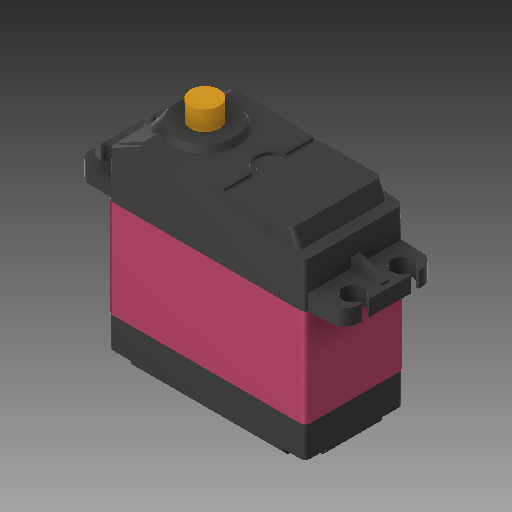
# Autodesk Inventor part: DS3218MG
Saved by Autodesk Inventor 2019.3 (Build 233278000, 278)
## iProperties
Created: 2019-03-07
Part Number: DS3218MG
Material: アルミニウム 6061
Document SubType Name: Modeling
Designer: TA
Density: 2.7 g/cm^3
Appearance: アルミニウム - フラット
Author: TA
Autodesk Inventor part; units mm, degrees
sketch "スケッチ1" plane through (0, 0, 0) normal (0, 1, 0) x (-1, 0, 0)
  line L0 (0, 0) -> (-40.06, 0)
  line L1 (-40.06, 0) -> (-40.06, -20)
  line L2 (-40.06, -20) -> (0, -20)
  line L3 (0, -20) -> (0, 0)
  dimension "d0" = 40.06
  dimension "d1" = 20
  constraints: 8 end point, 2 parallel, 1 horizontal, 1 perpendicular
  measures "d0" distance of L2.end L1.end
  measures "d1" distance of L1.end L0.end
ref_plane "作業平面1" through (0, 7.8, 0) normal (0, 1, 0) x (-1, 0, 0)
sketch "スケッチ2" plane through (0, 7.8, 0) normal (0, 1, 0) x (-1, 0, 0)
  line L0 (0.07, -20.1) -> (-40.13, -20.1)
  line L1 (-40.13, -20.1) -> (-40.13, 0.1)
  line L2 (-40.13, 0.1) -> (0.07, 0.1)
  line L3 (0.07, 0.1) -> (0.07, -20.1)
  line L4 (-40.06, -20) -> (0, -20) construction
  line L5 (0, -20) -> (0, 0) construction
  line L6 (0, 0) -> (-40.06, 0) construction
  line L7 (-40.06, 0) -> (-40.06, -20) construction
  dimension "d3" = 20.2
  dimension "d5" = 0.1
  dimension "d6" = 40.2
  dimension "d7" = 0.07
  constraints: 8 end point, 2 parallel, 1 horizontal, 1 perpendicular
  measures "d3" distance of L0.end L1.end
  measures "d5" distance between parallel lines of L0 L4
  measures "d6" distance of L1.end L2.end
  measures "d7" distance between parallel lines of L3 L5
loft "ロフト1" add profiles "スケッチ1", "スケッチ2"
fillet "フィレット2" radius 1 4 edges at (-0.035, 3.9, 0.05) (40.095, 3.9, 0.05) (40.095, 3.9, -20.05) (-0.035, 3.9, -20.05)
sketch "スケッチ4" plane through (0.9999, 0, -20) normal (0, -1, 0) x (1, 0, 0)
  line L0 (-1.0699, 15.5) -> (3.5301, 15.5)
  line L1 (3.5301, 15.5) -> (3.5301, 20.1)
  ellipse E0 centre (-0.0699, 19.0999) end of major axis (-0.6434, 19.9193) minor radius 1 (-0.07, 20.1) -> (-1.0699, 19.1) ccw projected
  line L2 (-0.07, 20.1) -> (38.1301, 20.1) projected
  line L3 (-1.0699, 0.9) -> (-1.0699, 19.1) projected
  point P0 (-0.9999, 20)
  dimension "d16" = 4.6
  dimension "d17" = 4.6
  constraints: 4 end point, 2 point on line, 1 perpendicular, 1 vertical, 1 other
  measures "d16" distance of L0.end L1.end
  measures "d17" distance between parallel lines of L3 L1
extrude "押し出し1" cut sketch "スケッチ4" against normal blind 1.5
fillet "フィレット3" radius 1.5 1 edges at (4.53, 0.75, -4.5)
ref_plane "作業平面2" through (0.9299, -780, -10) normal (0, 0, 1) x (-1, 0, 0)
ref_plane "作業平面3" through (20.03, -2231.9143, -19.1) normal (-1, 0, 0) x (0, 0, -1)
mirror "ミラー1" about plane through (0.9299, -780, -10) normal (0, 0, 1) of "押し出し1"
mirror "ミラー2" about plane through (20.03, -2231.9143, -19.1) normal (-1, 0, 0) of "押し出し1", "ミラー1"
chamfer "面取り1" distance 1 angle 45 4 edges at (20.03, 0, 0) (0, 0, -10) (20.03, 0, -20) (40.06, 0, -10)
sketch "スケッチ5" plane through (0.9299, 7.8, 0.1) normal (0, 1, 0) x (1, 0, 0)
  ellipse E0 centre (0.0001, 19.1999) end of major axis (-0.5734, 20.0193) minor radius 1 (0, 20.2) -> (-0.9999, 19.2) ccw projected
  line L0 (-0.9999, 19.2) -> (-0.9999, 1) projected
  ellipse E1 centre (0.0001, 1.0001) end of major axis (-0.5734, 0.1807) minor radius 1 (-0.9999, 1) -> (0, 0) ccw projected
  line L1 (0, 0) -> (38.2001, 0) projected
  ellipse E2 centre (38.2, 1.0001) end of major axis (38.7736, 0.1807) minor radius 1 (38.2001, 0) -> (39.2001, 1) ccw projected
  line L2 (39.2001, 1) -> (39.2001, 19.2) projected
  ellipse E3 centre (38.2, 19.1999) end of major axis (38.7736, 20.0193) minor radius 1 (39.2001, 19.2) -> (38.2001, 20.2) ccw projected
  line L3 (38.2001, 20.2) -> (0, 20.2) projected
  point P0 (-0.9299, 0.1)
  constraints: 4 other
extrude "押し出し2" add sketch "スケッチ5" along normal blind 19.9 separate body
sketch "スケッチ6" plane through (0.9299, 27.7, 0.1) normal (0, 1, 0) x (1, 0, 0)
  ellipse E0 centre (0.0001, 19.1999) end of major axis (-0.5734, 20.0193) minor radius 1 (0, 20.2) -> (-0.9999, 19.2) ccw projected
  line L0 (-0.9999, 19.2) -> (-0.9999, 1) projected
  ellipse E1 centre (0.0001, 1.0001) end of major axis (-0.5734, 0.1807) minor radius 1 (-0.9999, 1) -> (0, 0) ccw projected
  line L1 (0, 0) -> (38.2001, 0) projected
  ellipse E2 centre (38.2, 1.0001) end of major axis (38.7736, 0.1807) minor radius 1 (38.2001, 0) -> (39.2001, 1) ccw projected
  line L2 (39.2001, 1) -> (39.2001, 19.2) projected
  ellipse E3 centre (38.2, 19.1999) end of major axis (38.7736, 20.0193) minor radius 1 (39.2001, 19.2) -> (38.2001, 20.2) ccw projected
  line L3 (38.2001, 20.2) -> (0, 20.2) projected
  point P0 (-0.9299, 0.1)
  constraints: 4 other
ref_plane "作業平面4" through (0.9299, 40.4, 0.1) normal (0, 1, 0) x (1, 0, 0)
sketch "スケッチ7" plane through (0.9299, 40.4, 0.1) normal (0, 1, 0) x (1, 0, 0)
  ellipse E0 centre (0.0001, 19.1999) end of major axis (-0.5734, 20.0193) minor radius 1 (0, 20.2) -> (-0.9999, 19.2) ccw projected
  line L0 (-0.9999, 19.2) -> (-0.9999, 1) construction
  ellipse E1 centre (0.0001, 1.0001) end of major axis (-0.5734, 0.1807) minor radius 1 (-0.9999, 1) -> (0, 0) ccw projected
  line L1 (0, 0) -> (38.2001, 0) construction
  ellipse E2 centre (38.2, 1.0001) end of major axis (38.7736, 0.1807) minor radius 1 (38.2001, 0) -> (39.2001, 1) ccw projected
  line L2 (39.2001, 1) -> (39.2001, 19.2) construction
  ellipse E3 centre (38.2, 19.1999) end of major axis (38.7736, 20.0193) minor radius 1 (39.2001, 19.2) -> (38.2001, 20.2) ccw projected
  line L3 (38.2001, 20.2) -> (0, 20.2) construction
  line L4 (0.1501, 20.025) -> (38.0501, 20.025)
  line L5 (39.0501, 19.025) -> (39.0501, 1.175)
  line L6 (38.0501, 0.175) -> (0.1501, 0.175)
  line L7 (-0.8499, 1.175) -> (-0.8499, 19.025)
  arc A0 (0.1501, 20.025) -> (-0.8499, 19.025) centre (0.1501, 19.025) ccw
  arc A1 (39.0501, 19.025) -> (38.0501, 20.025) centre (38.0501, 19.025) ccw
  arc A2 (-0.8499, 1.175) -> (0.1501, 0.175) centre (0.1501, 1.175) ccw
  arc A3 (38.0501, 0.175) -> (39.0501, 1.175) centre (38.0501, 1.175) ccw
  point P0 (-0.9299, 0.1)
  point P1 (39.0501, 0.175)
  point P2 (39.0501, 20.025)
  point P3 (-0.8499, 0.175)
  dimension "d29" = 1.0001
  dimension "d27" = 39.9
  dimension "d28" = 19.85
  dimension "d30" = 1
  dimension "d31" = 40.2
  dimension "d32" = 0.15
  dimension "d33" = 0.175
  dimension "d34" = 20.2
  dimension "d35" = 1
  constraints: 8 end point, 8 point on circle, 8 tangent, 6 point on line, 4 centre point, 2 equal radius, 2 parallel, 1 horizontal, 1 perpendicular, 4 other
  measures "d27" distance of point (39.05, 0.175) point (-0.85, 0.175)
  measures "d28" distance of point (39.05, 20.025) point (39.05, 0.175)
  measures "d30" radius of A0
  measures "d31" distance between parallel lines of L2 L0
  measures "d32" distance between parallel lines of L2 L5
  measures "d33" distance between parallel lines of L3 L4
  measures "d34" distance between parallel lines of L3 L1
  measures "d35" radius of A1
loft "ロフト2" add profiles "スケッチ6", "スケッチ7" separate body
sketch "スケッチ8" plane through (0, 0, 0) normal (0, 0, 1) x (1, 0, 0)
  line L0 (0, 36.7) -> (6.3, 40)
  line L1 (1.08, 40.4) -> (38.98, 40.4) projected
  line L2 (38.98, 40.4) -> (0, 40.4)
  line L3 (0, 40.4) -> (0, 36.7)
  line L4 (39.1301, 27.7) -> (40.13, 27.7) projected
  line L5 (40.13, 27.7) -> (39.98, 40.4) projected
  line L6 (38.98, 40.4) -> (39.98, 40.4) projected
  line L7 (39.1301, 27.7) -> (38.98, 40.4) projected
  line L8 (38.98, 40.4) -> (1.08, 40.4) projected
  line L9 (16.63, 40) -> (40.0225, 36.8)
  line L10 (40.13, 27.7) -> (39.98, 40.4) projected
  line L11 (40.0225, 36.8) -> (39.98, 40.4)
  line L12 (39.98, 40.4) -> (13.1688, 40.4)
  line L13 (6.3, 40) -> (16.63, 40)
  point P0 (0, 0)
  dimension "d43" = 3.7
  dimension "d44" = 3.6
  dimension "d45" = 0.4
  dimension "d46" = 6.3
  dimension "d47" = 23.5
  constraints: 14 end point, 4 point on line, 2 horizontal, 1 collinear, 1 parallel, 1 perpendicular
  measures "d43" distance of L2.end L0.start
  measures "d44" distance from line of L1 L9.end
  measures "d45" distance between parallel lines of L13 L1
  measures "d46" distance from line of L0.end L3
  measures "d47" horizontal distance of L9.start L4.end
extrude "押し出し3" cut sketch "スケッチ8" against normal through all contours L3 L2 L1 L7 L9 L13 L0 | L7 L6 L5 L9 bodies 3
ref_plane "作業平面5" through (6.3, 40.4, -19.9305) normal (0, 1, 0) x (1, 0, 0)
sketch "スケッチ9" plane through (6.3, 40.4, -19.9305) normal (0, 1, 0) x (1, 0, 0)
  line L0 (-5.6775, -0.8055) -> (31.6225, -0.8055)
  line L1 (31.6225, -0.8055) -> (31.6225, -19.0555)
  line L2 (31.6225, -19.0555) -> (-5.6775, -19.0555)
  line L3 (-5.6775, -19.0555) -> (-5.6775, -0.8055)
  line L4 (33.7225, -0.9559) -> (33.7225, -18.9051) projected
  line L5 (-6.2635, -18.9062) -> (-6.2635, -0.9548) projected
  line L6 (32.7209, -19.9032) -> (10.33, -19.861) projected
  line L7 (10.33, 0) -> (32.7209, 0.0422) projected
  line L8 (-5.6775, -9.9305) -> (31.6225, -9.9305) construction
  line L9 (32.8301, 0.1695) -> (-5.3701, 0.1695) construction
  line L10 (-5.3701, -20.0305) -> (32.8301, -20.0305) construction
  point P0 (-6.3, -19.9305)
  dimension "d49" = 18.25
  dimension "d50" = 37.3
  dimension "d51" = 2.1
  dimension "d52" = 0.586
  dimension "d53" = 39.986
  dimension "d56" = 0.975
  dimension "d57" = 20.2
  constraints: 10 end point, 2 midpoint, 2 parallel, 1 horizontal, 1 perpendicular
  measures "d49" distance of L0.end L1.end
  measures "d50" distance between parallel lines of L1 L3
  measures "d51" distance between parallel lines of L4 L1
  measures "d52" distance between parallel lines of L3 L5
  measures "d53" distance between parallel lines of L4 L5
  measures "d56" distance between parallel lines of L0 L9
  measures "d57" distance between parallel lines of L10 L9
extrude "押し出し4" add sketch "スケッチ9" against normal blind 5 bodies 3
sketch "スケッチ10" plane through (0.6225, 40.4, -0.875) normal (0, 0, 1) x (1, 0, 0)
  line L0 (0, 0) -> (0, -3.3739) projected
  line L1 (0, -2.9224) -> (5.5791, 0)
  line L2 (37.3, 0) -> (0, 0) projected
  line L3 (5.6775, -0.4) -> (0.4202, -3.1538) projected
  line L4 (38.3984, -3.463) -> (16.0075, -0.4) projected
  line L5 (37.3, -3.3127) -> (35.9075, 0)
  line L6 (35.9075, 0) -> (37.3, 0)
  line L7 (37.3, 0) -> (37.3, -3.3127) projected
  line L8 (37.3, -3.3127) -> (37.3, 0)
  line L9 (39.5075, -32.6) -> (39.5075, -12.7) projected
  line L10 (0, -2.9224) -> (0, 0)
  line L11 (0, 0) -> (5.5791, 0)
  point P0 (-0.6225, -40.4)
  dimension "d61" = 3.6
  dimension "d62" = 0.4
  constraints: 12 end point, 4 collinear, 4 point on line, 1 parallel
  measures "d61" distance from line of L9 L5.end
  measures "d62" distance between parallel lines of L1 L3
extrude "押し出し5" cut sketch "スケッチ10" against normal through all bodies 3
fillet "フィレット4" radius 1.5 5 edges at (6.2016, 40.4, -10) (6.3, 40, -0.4722) (6.3, 40, -19.5278) (16.63, 40, -0.4722) (16.63, 40, -19.5278)
fillet "フィレット4" radius 1 4 edges at (0.6225, 37.2519, -0.875) (0.6225, 37.2519, -19.125) (37.2263, 38.7436, -0.875) (37.2263, 38.7436, -19.125)
ref_plane "作業平面6" through (0.9299, 7.8, -10) normal (0, 0, 1) x (1, 0, 0)
ref_plane "作業平面7" through (9.63, 7.8, -19.1) normal (-1, 0, 0) x (0, 0, 1)
sketch "スケッチ11" plane through (0.9299, 7.8, -10) normal (0, 0, 1) x (1, 0, 0)
  line L0 (8.7001, -15.88) -> (8.7001, 40.68) construction
  line L1 (34.5153, 32.6) -> (35.8417, 29.4447) construction
  line L2 (34.5153, 32.6) -> (5.6407, 32.6) construction
  arc A0 (5.6407, 32.6) -> (4.9447, 32.4287) centre (5.6407, 31.1) ccw construction
  line L3 (4.9447, 32.4287) -> (0.6926, 30.2014) construction
  line L4 (0.6926, 29.7499) -> (0.6926, 30.2014) construction
  line L5 (5.0431, 32.0287) -> (0.6926, 29.7499) construction
  arc A1 (5.7391, 32.2) -> (5.0431, 32.0287) centre (5.7391, 30.7) ccw construction
  line L6 (15.598, 32.2) -> (5.7391, 32.2) construction
  arc A2 (15.8013, 32.1862) -> (15.598, 32.2) centre (15.598, 30.7) ccw construction
  line L7 (35.8417, 29.4447) -> (15.8013, 32.1862) construction
  line L8 (0.6926, 30.2014) -> (-0.3074, 29.6776) construction
  line L9 (-0.3074, 29.6776) -> (-0.3074, 29.2261) construction
  line L10 (-0.3074, 29.2261) -> (0.6926, 29.7499) construction
  line L11 (0.6926, 29.7499) -> (0.6926, 30.2014) construction
  line L12 (8.7001, 33.5851) -> (2.7001, 33.5851)
  line L13 (-0.3074, 29.6776) -> (-0.3074, 29.2261) projected
  line L14 (2.7001, 33.5851) -> (-0.3074, 29.6776)
  line L15 (-0.3074, 29.6776) -> (0.6926, 30.2014) projected
  line L16 (-0.3074, 29.6776) -> (8.7001, 29.6776)
  line L17 (8.7001, 29.6776) -> (8.7001, 33.5851)
  point P0 (-0.9299, -7.8)
  dimension "d68" = 6
  constraints: 8 end point, 2 perpendicular, 2 point on line, 1 horizontal
  measures "d68" distance of L12.start L12.end
revolve "回転1" add sketch "スケッチ11" angle 360 about axis through (9.63, 7.8, -10) along (0, 1, 0) bodies 2
sketch "スケッチ12" plane through (6.3, 40.4, -19.9305) normal (0, 1, 0) x (1, 0, 0)
  line L0 (17.43, -19.0555) -> (17.43, -12.9899)
  arc A0 (17.0106, -7.3646) -> (17.0106, -12.4965) centre (17.43, -9.9305) ccw
  ellipse E0 centre (29.1452, -1.8055) end of major axis (30.23, -1.8055) minor radius 1 (30.23, -1.8055) -> (29.1452, -0.8055) ccw construction
  line L1 (0.2707, -0.8055) -> (29.1452, -0.8055) construction
  line L2 (0.2707, -19.0555) -> (0.2707, -0.8055) construction
  line L3 (29.1452, -19.0555) -> (0.2707, -19.0555) construction
  ellipse E1 centre (29.1452, -18.0555) end of major axis (30.23, -18.0555) minor radius 1 (29.1452, -19.0555) -> (30.23, -18.0555) ccw construction
  line L4 (30.23, -18.0555) -> (30.23, -1.8055) construction
  line L5 (17.43, -6.8711) -> (17.43, -0.8055)
  line L6 (10.4312, -0.8055) -> (30.4716, -0.8055) construction
  line L7 (16.43, -19.0555) -> (16.43, -13.3888)
  arc A1 (16.43, -6.4722) -> (16.43, -13.3888) centre (17.43, -9.9305) ccw
  line L8 (16.43, -6.4722) -> (16.43, -0.8055)
  line L9 (16.43, -19.0555) -> (17.43, -19.0555)
  line L10 (-1.77, -18.9305) -> (29.23, -18.9305) projected
  line L11 (16.43, -0.8055) -> (17.43, -0.8055)
  arc A2 (17.0106, -7.3646) -> (17.43, -6.8711) centre (16.93, -6.8711) ccw
  arc A3 (17.43, -12.9899) -> (17.0106, -12.4965) centre (16.93, -12.9899) ccw
  point P0 (-6.3, -19.9305)
  point P1 (17.43, -12.5305)
  point P2 (17.43, -7.3305)
  dimension "d70" = 5.2
  dimension "d71" = 12.8
  dimension "d72" = 0
  dimension "d73" = 1
  dimension "d74" = 0.5
  constraints: 12 end point, 10 point on circle, 4 centre point, 4 point on line, 4 tangent, 3 collinear, 2 parallel, 1 equal radius, 1 perpendicular, 1 vertical, 4 other
  measures "d70" diameter of A0
  measures "d71" distance between parallel lines of L4 L5
  measures "d72" distance from line of L5 A0.centre
  measures "d73" distance between parallel lines of L0 L7
  measures "d74" radius of A2
extrude "押し出し6" cut sketch "スケッチ12" against normal blind 0.5 bodies 3
sketch "スケッチ13" plane through (9.63, 41.3851, -10) normal (0, 1, 0) x (1, 0, 0)
  circle A0 centre (0, 0) radius 2.95
  point P0 (-9.63, -10)
  dimension "d77" = 5.9
  constraints: 1 centre point
  measures "d77" diameter of A0
extrude "押し出し7" add sketch "スケッチ13" along normal blind 4 bodies 2
sketch "スケッチ14" plane through (0.9299, 27.7, -20.1) normal (0, -1, 0) x (1, 0, 0)
  ellipse E0 centre (0.0001, 1.0001) end of major axis (-0.5734, 0.1807) minor radius 1 (-0.9999, 1) -> (0, 0) ccw construction
  ellipse E1 centre (0.0001, 19.1999) end of major axis (-0.5734, 20.0193) minor radius 1 (0, 20.2) -> (-0.9999, 19.2) ccw construction
  ellipse E2 centre (0.0001, 1.0001) end of major axis (-0.5734, 0.1807) minor radius 1 (-0.9999, 1) -> (0, 0) ccw construction
  line L0 (-0.9367, 0.65) -> (-8.2367, 0.85)
  line L1 (-8.2367, 0.85) -> (-8.2367, 19.35)
  line L2 (-8.2367, 19.35) -> (-0.9367, 19.55)
  line L3 (-0.9367, 0.65) -> (-0.9367, 19.55)
  line L4 (-0.9367, 0.65) -> (-0.4098, 0.65)
  line L5 (-0.4098, 0.65) -> (-0.4098, 19.5644)
  line L6 (-0.4098, 19.5644) -> (-0.9367, 19.55)
  dimension "d5" = 0.1
  dimension "d83" = 18.9
  dimension "d84" = 7.3
  dimension "d85" = 18.5
  constraints: 14 end point, 3 vertical, 1 collinear, 1 equal length, 1 horizontal, 5 other
  measures "d83" distance of L0.start L2.end
  measures "d84" distance between parallel lines of L1 L3
  measures "d85" distance of L0.end L1.end
extrude "押し出し8" add sketch "スケッチ14" against normal blind 3.2 bodies 3
fillet "フィレット5" radius 3 2 edges at (-7.3068, 29.3, -0.75) (-7.3068, 29.3, -19.25)
sketch "スケッチ15" plane through (0.9299, 30.9, -20.1) normal (0, 1, 0) x (1, 0, 0)
  line L0 (-5.6499, -5.1) -> (-5.6499, -15.1) construction
  line L1 (-8.2367, -3.7689) -> (-8.2367, -16.4311) construction
  line L2 (-8.2367, -10.1) -> (-2.6661, -10.1) construction
  line L3 (19.1001, -24.2414) -> (19.1001, 4.0414) projected
  point P0 (-0.9299, -20.1)
  dimension "d89" = 10
  dimension "d97" = 5
  dimension "d98" = 24.75
  constraints: 4 end point, 1 horizontal, 1 midpoint, 1 vertical
  measures "d89" distance of L0.start L0.end
  measures "d97" distance from line of L0.end L2
  measures "d98" distance from line of L3 L0.end
hole "穴1" at (-4.72, 30.9, -15) at (-4.72, 30.9, -5) direction (0, -1, 0) diameter 4.3 end through all bodies 3
ref_plane "作業平面8" through (20.03, 1729.5, -18.9757) normal (-1, 0, 0) x (0, 0, 1)
sketch "スケッチ16" plane through (0.9299, 30.9, -20.1) normal (0, 1, 0) x (1, 0, 0)
  line L0 (-8.5257, -4.35) -> (-7.5257, -4.35)
  line L1 (-7.5257, -4.35) -> (-7.5257, -5.85)
  line L2 (-7.5257, -5.85) -> (-8.5257, -5.85)
  line L3 (-8.5257, -5.85) -> (-8.5257, -4.35)
  circle A0 centre (-5.6499, -5.1) radius 2.15 construction
  circle A1 centre (-5.6499, -15.1) radius 2.15 construction
  arc A2 (-5.3189, -0.7701) -> (-8.2367, -3.7689) centre (-5.2367, -3.7689) ccw construction
  line L4 (-8.2367, -3.7689) -> (-8.2367, -16.4311) construction
  arc A3 (-8.2367, -16.4311) -> (-5.3189, -19.4299) centre (-5.2367, -16.4311) ccw construction
  line L5 (-5.3189, -19.4299) -> (-0.8806, -19.5515) construction
  line L6 (-0.9621, -1.0441) -> (-0.9621, -19.1559) construction
  line L7 (-0.8812, -0.65) -> (-0.9367, -0.65) construction
  line L8 (-0.9367, -0.65) -> (-5.3189, -0.7701) construction
  point P0 (-0.9299, -20.1)
  dimension "d99" = 1
  dimension "d100" = 1.5
  dimension "d101" = 0.75
  constraints: 8 end point, 2 parallel, 1 horizontal, 1 perpendicular, 2 other
  measures "d99" distance of L1.end L2.end
  measures "d100" distance of L0.end L1.end
  measures "d101" distance from line of L0 A0.centre
extrude "押し出し9" cut sketch "スケッチ16" against normal through all bodies 3
ref_plane "作業平面9" through (-344.9318, 27.7, -10) normal (0, 0, 1) x (0, 1, 0)
mirror "ミラー4" about plane through (-344.9318, 27.7, -10) normal (0, 0, 1) of "押し出し9" bodies 3
sketch "スケッチ17" plane through (-344.9318, 27.7, -10) normal (0, 0, 1) x (0, 1, 0)
  line L0 (3.2, -340.5428) -> (3.2, -344.9811) projected
  line L1 (3.2, -344.8996) -> (9.0191, -344.9683) projected
  line L2 (3.2, -337.625) -> (3.2, -340.5428) projected
  line L3 (3.2, -338.6996) -> (3.7, -338.6996)
  line L4 (3.7, -338.6996) -> (5.2, -343.9232)
  line L5 (5.2, -343.9232) -> (5.2, -344.9232)
  line L6 (3.2, -344.8996) -> (9.0191, -344.9683) projected
  point P0 (-27.7, -344.9318)
  dimension "d104" = 6.2
  dimension "d105" = 2
  dimension "d106" = 0.5
  dimension "d107" = 1
  constraints: 6 end point, 2 point on line, 1 horizontal, 1 perpendicular
  measures "d104" distance from line of L1.start L3
  measures "d105" distance between parallel lines of L0 L5
  measures "d106" distance of L3.start L3.end
  measures "d107" distance of L4.end L5.end
extrude "押し出し10" add sketch "スケッチ17" along normal mid plane 1.63 bodies 3
sketch "スケッチ18" plane through (-0.07, 7.8, -19.1) normal (-1, 0, 0) x (0, 0, 1)
  line L0 (14.6, -6.8) -> (3.6, -6.8) projected
  line L1 (14.6, -6.8) -> (14.6, -6.3) projected
  line L2 (14.6, -6.3) -> (18.1193, -6.3) projected
  line L3 (18.2001, 0) -> (18.1193, -6.3) projected
  line L4 (0, 0) -> (18.2001, 0) projected
  line L5 (0.0808, -6.3) -> (0, 0) projected
  line L6 (0.0808, -6.3) -> (3.6, -6.3) projected
  line L7 (3.6, -6.3) -> (3.6, -6.8) projected
  line L8 (5.65, 0) -> (12.55, 0)
  line L9 (12.55, 0) -> (12.55, -4.5)
  line L10 (12.55, -4.5) -> (5.65, -4.5)
  line L11 (5.65, -4.5) -> (5.65, 0)
  point P0 (19.1, -7.8)
  dimension "d110" = 6.9
  dimension "d111" = 4.5
  dimension "d112" = 18.2001
  dimension "d113" = 5.65
  constraints: 8 end point, 2 parallel, 1 horizontal, 1 perpendicular, 1 point on line
  measures "d110" distance of L9.end L10.end
  measures "d111" distance of L8.end L9.end
  measures "d112" distance of L4.start L3.start
  measures "d113" distance from line of L3.start L9
extrude "押し出し11" add sketch "スケッチ18" along normal blind 6 and the other way blind 1 separate body contours L9 L10 L11 L4
mirror "ミラー6" about plane through (20.03, 1729.5, -18.9757) normal (-1, 0, 0) of "押し出し10", "穴1", "フィレット5", "押し出し8", "押し出し9", "ミラー4" bodies 3
equation "\"d5\" = -0.5 * d1 + 0.5 * d3"
equation "\"d7\" = -0.5 * d0 + 0.5 * d6"
equation "\"d32\" = -0.5 * d27 + 0.5 * d31"
equation "\"d33\" = -0.5 * d28 + 0.5 * d34"
equation "\"d56\" = -0.5 * d49 + 0.5 * d57"
equation "\"d97\" = 0.5 * d89"
equation "\"d101\" = 0.5 * d100"
equation "\"d113\" = -0.5 * d110 + 0.5 * d112"
